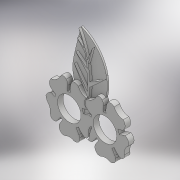
# Autodesk Inventor part: RosaV2
Saved by Autodesk Inventor 2017 (Build 210142000, 142)
## iProperties
Created: 2018-06-14
Part Number: RosaV2
Material: Generic
Document SubType Name: Modeling
Designer: Carolina Lema
Density: 1 g/cm^3
Appearance: Default
Author: Carolina Lema
Autodesk Inventor part; units mm, degrees
ref_plane "YZ Plane" through (0, 0, 0) normal (1, 0, 0) x (0, 1, 0)
ref_plane "XZ Plane" through (0, 0, 0) normal (0, 1, 0) x (-1, 0, 0)
ref_plane "XY Plane" through (0, 0, 0) normal (0, 0, 1) x (1, 0, 0)
sketch "Sketch1" plane through (0, 0, 0) normal (0, 1, 0) x (-1, 0, 0)
  arc A0 (-50.2935, -141.9625) -> (-50.5085, -138.2118) centre (-57.4787, -140.493) ccw
  arc A1 (-49.4604, -134.8668) -> (-50.5085, -138.2118) centre (-45.5145, -137.94) ccw
  arc A2 (-52.2706, -141.9093) -> (-53.5294, -134.3132) centre (-66.0628, -140.2926) ccw
  arc A3 (-60.8507, -147.4866) -> (-64.2809, -146.6761) centre (-66.0428, -161.7965) ccw
  circle A4 centre (-51.5636, -152.3854) radius 8.5
  arc A5 (-45.2271, -160.758) -> (-42.1345, -164.9104) centre (-15.6123, -141.9291) ccw
  arc A6 (-38.966, -164.9101) -> (-37.6707, -160.6686) centre (-43.0606, -161.3412) ccw
  arc A7 (-44.5421, -165.2935) -> (-46.8275, -161.7567) centre (-172.1244, -245.2288) ccw
  arc A8 (-37.8657, -145.4277) -> (-38.2191, -140.1494) centre (-41.6996, -143.0334) ccw
  arc A9 (-45.6096, -134.3885) -> (-38.2191, -140.1494) centre (-36.6467, -130.5112) ccw
  arc A10 (-36.1368, -156.274) -> (-37.6707, -160.6686) centre (-32.4682, -160.0194) ccw
  arc A11 (-36.1368, -156.274) -> (-34.6048, -152.385) centre (-42.1305, -151.6666) ccw
  arc A12 (-41.3682, -149.8747) -> (-38.503, -148.5121) centre (-47.6774, -132.9147) ccw
  arc A13 (-41.9398, -148.1863) -> (-37.8657, -145.4277) centre (-47.8277, -135.103) ccw
  arc A14 (-34.6048, -152.385) -> (-38.503, -148.5121) centre (-40.8573, -154.78) ccw
  arc A15 (-63.8657, -139.5775) -> (-58.174, -134.8668) centre (-65.1246, -132.2626) ccw
  arc A16 (-53.5294, -134.3132) -> (-58.174, -134.8668) centre (-55.4761, -137.7415) ccw
  arc A17 (-45.6096, -134.3885) -> (-49.4604, -134.8668) centre (-47.2959, -136.5525) ccw
  line L0 (-46.3394, -171.0352) -> (-46.3407, -171.0345)
  arc A18 (-48.8902, -170.6862) -> (-44.9412, -169.507) centre (-47.5666, -167.9168) ccw
  arc A19 (-65.6657, -161.3497) -> (-62.9245, -164.9101) centre (-62.7518, -161.9418) ccw
  arc A20 (-62.9245, -164.9101) -> (-58.2423, -160.4876) centre (-68.2851, -154.5449) ccw
  arc A21 (-56.5584, -161.6213) -> (-58.6246, -165.2834) centre (21.5695, -208.1162) ccw
  arc A22 (-58.6246, -165.2834) -> (-59.26, -166.6979) centre (-55.3426, -167.6077) ccw
  arc A23 (-59.26, -166.6979) -> (-53.816, -170.3276) centre (-55.8552, -167.4887) ccw
  arc A24 (-48.8902, -170.6862) -> (-53.816, -170.3276) centre (-51.7693, -176.2225) ccw
  arc A25 (-65.6657, -161.3497) -> (-67.4979, -155.3741) centre (-72.0774, -160.047) ccw
  arc A26 (-61.8781, -150.4206) -> (-66.2243, -148.9882) centre (-82.2432, -204.906) ccw
  arc A27 (-42.1345, -164.9104) -> (-38.966, -164.9101) centre (-40.5505, -161.8463) ccw
  arc A28 (-44.9412, -169.507) -> (-44.5421, -165.2935) centre (-48.2055, -167.0721) ccw
  arc A29 (-76.2935, -141.9625) -> (-76.5085, -138.2118) centre (-83.4787, -140.493) ccw
  arc A30 (-75.4604, -134.8668) -> (-76.5085, -138.2118) centre (-71.5145, -137.94) ccw
  arc A31 (-78.2706, -141.9093) -> (-79.5294, -134.3132) centre (-92.0628, -140.2926) ccw
  arc A32 (-86.8507, -147.4866) -> (-90.2809, -146.6761) centre (-92.0428, -161.7965) ccw
  circle A33 centre (-77.5636, -152.3854) radius 8.5
  arc A34 (-71.2271, -160.758) -> (-68.1345, -164.9104) centre (-41.6123, -141.9291) ccw
  arc A35 (-70.5421, -165.2935) -> (-72.8275, -161.7567) centre (-198.1244, -245.2288) ccw
  arc A36 (-63.8657, -145.4277) -> (-64.2191, -140.1494) centre (-67.6996, -143.0334) ccw
  arc A37 (-71.6096, -134.3885) -> (-64.2191, -140.1494) centre (-62.6467, -130.5112) ccw
  arc A38 (-67.9398, -148.1863) -> (-63.8657, -145.4277) centre (-73.8277, -135.103) ccw
  arc A39 (-90.7671, -139.6764) -> (-84.174, -134.8668) centre (-91.1246, -132.2626) ccw
  arc A40 (-79.5294, -134.3132) -> (-84.174, -134.8668) centre (-81.4761, -137.7415) ccw
  arc A41 (-71.6096, -134.3885) -> (-75.4604, -134.8668) centre (-73.2959, -136.5525) ccw
  line L1 (-72.3394, -171.0352) -> (-72.3407, -171.0345)
  arc A42 (-74.8902, -170.6862) -> (-70.9412, -169.507) centre (-73.5666, -167.9168) ccw
  arc A43 (-91.6657, -161.3497) -> (-88.9245, -164.9101) centre (-88.7518, -161.9418) ccw
  arc A44 (-88.9245, -164.9101) -> (-84.2423, -160.4876) centre (-94.2851, -154.5449) ccw
  arc A45 (-82.5584, -161.6213) -> (-84.6246, -165.2834) centre (-4.4305, -208.1162) ccw
  arc A46 (-84.6246, -165.2834) -> (-85.26, -166.6979) centre (-81.3426, -167.6077) ccw
  arc A47 (-85.26, -166.6979) -> (-79.816, -170.3276) centre (-81.8552, -167.4887) ccw
  arc A48 (-74.8902, -170.6862) -> (-79.816, -170.3276) centre (-77.7693, -176.2225) ccw
  arc A49 (-91.6639, -144.9966) -> (-90.2809, -146.6761) centre (-87.4857, -142.9652) ccw
  arc A50 (-90.7671, -139.6764) -> (-91.6639, -144.9966) centre (-87.4857, -142.9652) ccw
  arc A51 (-91.6657, -161.3497) -> (-94.028, -154.908) centre (-98.0774, -160.047) ccw
  arc A52 (-92.2243, -148.9882) -> (-94.028, -154.908) centre (-90.5316, -152.7386) ccw
  arc A53 (-87.8781, -150.4206) -> (-92.2243, -148.9882) centre (-108.2432, -204.906) ccw
  arc A54 (-68.1345, -164.9104) -> (-64.966, -164.9101) centre (-66.5505, -161.8463) ccw
  arc A55 (-70.9412, -169.507) -> (-70.5421, -165.2935) centre (-74.2055, -167.0721) ccw
  arc A56 (-66.2243, -148.9882) -> (-67.3918, -149.7806) centre (-64.5316, -152.7386) ccw
  circle A57 centre (-51.5636, -152.3854) radius 10.5
  circle A58 centre (-77.5636, -152.3854) radius 10.5
  arc A59 (-66.5505, -161.8463) -> (-64.966, -164.9101) centre (-62.3299, -161.6052) ccw
  arc A60 (-66.5505, -161.8463) -> (-67.9398, -156.5846) centre (-74.2403, -161.0624) ccw
  arc A61 (-64.2809, -146.6761) -> (-63.8657, -139.5775) centre (-67.8597, -142.9054) ccw
  line L2 (-53.5294, -134.3132) -> (-53.5294, -99.3132)
  line L3 (-53.5294, -99.3132) -> (-75.4604, -134.8668)
  line L4 (-75.4604, -134.8668) -> (-75.4604, -99.3132)
  line L5 (-75.4604, -99.3132) -> (-53.5294, -134.3132)
  point P0 (0, 0)
  point P1 (-51.4803, -152.4063)
  point P2 (-45.3977, -162.821)
  point P3 (-45.3977, -141.9574)
  point P4 (-33.5868, -132.2626)
  point P5 (-34.505, -161.7965)
  point P6 (-36.7472, -154.5449)
  point P7 (-47.2742, -170.9723)
  point P8 (-57.8397, -162.8189)
  point P9 (-56.1478, -170.9718)
  point P10 (-71.3977, -162.821)
  point P11 (-71.3977, -141.9574)
  point P12 (-59.5868, -132.2626)
  point P13 (-60.505, -161.7965)
  point P14 (-62.7472, -154.5449)
  point P15 (-73.2742, -170.9723)
  point P16 (-83.8397, -162.8189)
  point P17 (-82.1478, -170.9718)
  dimension "d2" = 21
  dimension "d3" = 21
  dimension "d0" = 17
  dimension "d1" = 17
  dimension "d6" = 35
  constraints: 128 point on circle, 60 centre point, 12 end point, 7 tangent, 2 coincident, 2 vertical, 1 concentric, 26 other
  measures "d0" diameter of A4
  measures "d1" diameter of A33
  measures "d6" distance of L2.start L2.end
extrude "Extrusion1" add sketch "Sketch1" along normal blind 4 contours A0 A1 A17 A9 A8 A13 A57 | A57 | A57 A3 A61 A15 A16 A2 | A12 A14 A11 A10 A6 A27 A5 A57 | A57 A20 A19 A25 A58 A56 A26 | A41 A37 A36 A38 A58 A29 A30 | A7 A28 A18 A24 A23 A22 A21 A57 | A58 | A58 A32 A49 A50 A39 A40 A31 | A60 A59 A54 A34 A58 | A58 A44 A43 A51 A52 A53 | A35 A55 A42 A48 A47 A46 A45 A58
sketch "Sketch4" plane through (0, 4, 0) normal (0, 1, 0) x (1, 0, 0)
  arc A0 (52.0058, 121.0973) -> (57.4996, 99.146) centre (415.9824, 200.5268) ccw
  arc A1 (54.1227, 139.9616) -> (52.0058, 121.0973) centre (80.9093, 127.4048) ccw
  arc A2 (63.864, 144.3907) -> (54.1227, 139.9616) centre (61.5923, 136.46) ccw
  arc A3 (57.4996, 99.146) -> (75.7221, 121.0973) centre (46.6692, 126.6758) ccw
  arc A4 (75.7221, 121.0973) -> (73.6052, 139.9616) centre (46.8187, 127.4048) ccw
  arc A5 (73.6052, 139.9616) -> (63.864, 144.3907) centre (66.1356, 136.46) ccw
  arc A6 (57.4996, 99.146) -> (63.864, 144.3907) centre (0.6464, 130.2132) ccw
  arc A7 (57.4996, 99.146) -> (62.7337, 144.6303) centre (-13.0806, 130.3112) ccw
  line L0 (63.5682, 139.1315) -> (54.1233, 123.015)
  line L1 (54.1233, 123.015) -> (63.864, 136.0011)
  line L2 (63.864, 124.6213) -> (55.2722, 115.1963)
  line L3 (55.2722, 115.1963) -> (63.5682, 121.4909)
  line L4 (61.2764, 109.723) -> (56.3279, 105.9683)
  line L5 (56.3279, 105.9683) -> (61.8855, 112.0649)
  line L6 (63.864, 116.0357) -> (67.3014, 107.1278)
  line L7 (67.3014, 107.1278) -> (64.3376, 118.3436)
  line L8 (65.3957, 132.4478) -> (75.743, 123.0153)
  line L9 (75.743, 123.0153) -> (65.424, 129.0627)
  point P0 (0, 0)
  constraints: 27 point on circle, 20 end point, 8 centre point, 2 parallel, 2 perpendicular, 2 tangent
extrude "Extrusion3" add sketch "Sketch4" against normal blind 1.2 contours A1 A2 A7 L0 L1 L2 L3 L5 L4 A0 | A6 L6 L7 L9 L8 A5 A4 A3
sketch "Sketch5" plane through (0, 4, 0) normal (0, 1, 0) x (1, 0, 0)
  arc A0 (65.3957, 132.4478) -> (64.6812, 140.0625) centre (0.6464, 130.2132) ccw projected
  circle A1 centre (51.5636, 152.3854) radius 8.5 projected
  circle A2 centre (77.5636, 152.3854) radius 8.5 projected
  arc A3 (63.8657, 139.5775) -> (63.5237, 139.5103) centre (65.1246, 132.2626) ccw projected
  arc A4 (63.4423, 140.1643) -> (63.8657, 139.5775) centre (67.8597, 142.9054) ccw projected
  arc A5 (63.4423, 140.1643) -> (62.8183, 144.1746) centre (-13.0806, 130.3112) ccw projected
  arc A6 (64.2809, 146.6761) -> (62.8183, 144.1746) centre (67.8597, 142.9054) ccw projected
  arc A7 (60.8507, 147.4866) -> (64.2809, 146.6761) centre (66.0428, 161.7965) ccw projected
  arc A8 (60.8507, 147.4866) -> (61.8781, 150.4206) centre (51.5636, 152.3854) ccw projected
  arc A9 (61.8781, 150.4206) -> (66.2243, 148.9882) centre (82.2432, 204.906) ccw projected
  arc A10 (66.2243, 148.9882) -> (67.3918, 149.7806) centre (64.5316, 152.7386) ccw projected
  arc A11 (67.3918, 149.7806) -> (67.9398, 148.1863) centre (77.5636, 152.3854) ccw projected
  arc A12 (67.9398, 148.1863) -> (63.8657, 145.4277) centre (73.8277, 135.103) ccw projected
  arc A13 (63.8657, 145.4277) -> (64.2191, 140.1494) centre (67.6996, 143.0334) ccw projected
  arc A14 (64.6812, 140.0625) -> (64.2191, 140.1494) centre (62.6467, 130.5112) ccw projected
  arc A15 (65.3957, 132.4478) -> (64.6812, 140.0625) centre (0.6464, 130.2132) ccw projected
  line L0 (65.3957, 132.4478) -> (75.743, 123.0153) projected
  line L1 (75.743, 123.0153) -> (65.424, 129.0627) projected
  arc A16 (64.3376, 118.3436) -> (65.424, 129.0627) centre (0.6464, 130.2132) ccw projected
  line L2 (64.3376, 118.3436) -> (67.3014, 107.1278) projected
  line L3 (67.3014, 107.1278) -> (63.864, 116.0357) projected
  arc A17 (57.4996, 99.146) -> (63.864, 116.0357) centre (0.6464, 130.2132) ccw projected
  arc A18 (57.4996, 99.146) -> (75.7221, 121.0973) centre (46.6692, 126.6758) ccw projected
  arc A19 (75.7221, 121.0973) -> (75.4494, 134.8528) centre (46.8187, 127.4048) ccw projected
  arc A20 (75.4494, 134.8528) -> (75.4604, 134.8668) centre (73.2959, 136.5525) ccw projected
  arc A21 (75.4604, 134.8668) -> (76.5085, 138.2118) centre (71.5145, 137.94) ccw projected
  arc A22 (76.2935, 141.9625) -> (76.5085, 138.2118) centre (83.4787, 140.493) ccw projected
  arc A23 (76.2935, 141.9625) -> (78.2706, 141.9093) centre (77.5636, 152.3854) ccw projected
  arc A24 (78.2706, 141.9093) -> (79.5294, 134.3132) centre (92.0628, 140.2926) ccw projected
  arc A25 (79.5294, 134.3132) -> (84.174, 134.8668) centre (81.4761, 137.7415) ccw projected
  arc A26 (90.7671, 139.6764) -> (84.174, 134.8668) centre (91.1246, 132.2626) ccw projected
  arc A27 (90.7671, 139.6764) -> (90.2809, 146.6761) centre (87.4857, 142.9652) ccw projected
  arc A28 (86.8507, 147.4866) -> (90.2809, 146.6761) centre (92.0428, 161.7965) ccw projected
  arc A29 (86.8507, 147.4866) -> (87.8781, 150.4206) centre (77.5636, 152.3854) ccw projected
  arc A30 (87.8781, 150.4206) -> (92.2243, 148.9882) centre (108.2432, 204.906) ccw projected
  arc A31 (92.2243, 148.9882) -> (94.028, 154.908) centre (90.5316, 152.7386) ccw projected
  arc A32 (91.6657, 161.3497) -> (94.028, 154.908) centre (98.0774, 160.047) ccw projected
  arc A33 (91.6657, 161.3497) -> (88.9245, 164.9101) centre (88.7518, 161.9418) ccw projected
  arc A34 (88.9245, 164.9101) -> (84.2423, 160.4876) centre (94.2851, 154.5449) ccw projected
  arc A35 (84.2423, 160.4876) -> (82.5584, 161.6213) centre (77.5636, 152.3854) ccw projected
  arc A36 (82.5584, 161.6213) -> (84.6246, 165.2834) centre (4.4305, 208.1162) ccw projected
  arc A37 (84.6246, 165.2834) -> (85.26, 166.6979) centre (81.3426, 167.6077) ccw projected
  arc A38 (85.26, 166.6979) -> (79.816, 170.3276) centre (81.8552, 167.4887) ccw projected
  arc A39 (74.8902, 170.6862) -> (79.816, 170.3276) centre (77.7693, 176.2225) ccw projected
  arc A40 (74.8902, 170.6862) -> (70.9412, 169.507) centre (73.5666, 167.9168) ccw projected
  arc A41 (70.9412, 169.507) -> (70.5421, 165.2935) centre (74.2055, 167.0721) ccw projected
  arc A42 (70.5421, 165.2935) -> (72.8275, 161.7567) centre (198.1244, 245.2288) ccw projected
  arc A43 (72.8275, 161.7567) -> (71.2271, 160.758) centre (77.5636, 152.3854) ccw projected
  arc A44 (71.2271, 160.758) -> (68.1345, 164.9104) centre (41.6123, 141.9291) ccw projected
  arc A45 (68.1345, 164.9104) -> (64.966, 164.9101) centre (66.5505, 161.8463) ccw projected
  arc A46 (66.5505, 161.8463) -> (64.966, 164.9101) centre (62.3299, 161.6052) ccw projected
  arc A47 (66.5505, 161.8463) -> (67.9398, 156.5846) centre (74.2403, 161.0624) ccw projected
  arc A48 (67.9398, 156.5846) -> (67.4979, 155.3741) centre (77.5636, 152.3854) ccw projected
  arc A49 (65.6657, 161.3497) -> (67.4979, 155.3741) centre (72.0774, 160.047) ccw projected
  arc A50 (65.6657, 161.3497) -> (62.9245, 164.9101) centre (62.7518, 161.9418) ccw projected
  arc A51 (62.9245, 164.9101) -> (58.2423, 160.4876) centre (68.2851, 154.5449) ccw projected
  arc A52 (58.2423, 160.4876) -> (56.5584, 161.6213) centre (51.5636, 152.3854) ccw projected
  arc A53 (56.5584, 161.6213) -> (58.6246, 165.2834) centre (-21.5695, 208.1162) ccw projected
  arc A54 (58.6246, 165.2834) -> (59.26, 166.6979) centre (55.3426, 167.6077) ccw projected
  arc A55 (59.26, 166.6979) -> (53.816, 170.3276) centre (55.8552, 167.4887) ccw projected
  arc A56 (48.8902, 170.6862) -> (53.816, 170.3276) centre (51.7693, 176.2225) ccw projected
  arc A57 (48.8902, 170.6862) -> (44.9412, 169.507) centre (47.5666, 167.9168) ccw projected
  arc A58 (44.9412, 169.507) -> (44.5421, 165.2935) centre (48.2055, 167.0721) ccw projected
  arc A59 (44.5421, 165.2935) -> (46.8275, 161.7567) centre (172.1244, 245.2288) ccw projected
  arc A60 (46.8275, 161.7567) -> (45.2271, 160.758) centre (51.5636, 152.3854) ccw projected
  arc A61 (45.2271, 160.758) -> (42.1345, 164.9104) centre (15.6123, 141.9291) ccw projected
  arc A62 (42.1345, 164.9104) -> (38.966, 164.9101) centre (40.5505, 161.8463) ccw projected
  arc A63 (38.966, 164.9101) -> (37.6707, 160.6686) centre (43.0606, 161.3412) ccw projected
  arc A64 (36.1368, 156.274) -> (37.6707, 160.6686) centre (32.4682, 160.0194) ccw projected
  arc A65 (36.1368, 156.274) -> (34.6048, 152.385) centre (42.1305, 151.6666) ccw projected
  arc A66 (34.6048, 152.385) -> (38.503, 148.5121) centre (40.8573, 154.78) ccw projected
  arc A67 (41.3682, 149.8747) -> (38.503, 148.5121) centre (47.6774, 132.9147) ccw projected
  arc A68 (41.3682, 149.8747) -> (41.9398, 148.1863) centre (51.5636, 152.3854) ccw projected
  arc A69 (41.9398, 148.1863) -> (37.8657, 145.4277) centre (47.8277, 135.103) ccw projected
  arc A70 (37.8657, 145.4277) -> (38.2191, 140.1494) centre (41.6996, 143.0334) ccw projected
  arc A71 (45.6096, 134.3885) -> (38.2191, 140.1494) centre (36.6467, 130.5112) ccw projected
  arc A72 (45.6096, 134.3885) -> (49.4604, 134.8668) centre (47.2959, 136.5525) ccw projected
  arc A73 (49.4604, 134.8668) -> (50.5085, 138.2118) centre (45.5145, 137.94) ccw projected
  arc A74 (50.2935, 141.9625) -> (50.5085, 138.2118) centre (57.4787, 140.493) ccw projected
  arc A75 (50.2935, 141.9625) -> (52.2706, 141.9093) centre (51.5636, 152.3854) ccw projected
  arc A76 (52.2706, 141.9093) -> (52.7297, 136.4107) centre (66.0628, 140.2926) ccw projected
  arc A77 (52.7297, 136.4107) -> (52.0058, 121.0973) centre (80.9093, 127.4048) ccw projected
  arc A78 (52.0058, 121.0973) -> (57.4996, 99.146) centre (415.9824, 200.5268) ccw projected
  arc A79 (57.4996, 99.146) -> (61.2764, 109.723) centre (-13.0806, 130.3112) ccw projected
  line L4 (61.2764, 109.723) -> (56.3279, 105.9683) projected
  line L5 (56.3279, 105.9683) -> (61.8855, 112.0649) projected
  arc A80 (61.8855, 112.0649) -> (63.5682, 121.4909) centre (-13.0806, 130.3112) ccw projected
  line L6 (63.5682, 121.4909) -> (55.2722, 115.1963) projected
  line L7 (55.2722, 115.1963) -> (63.864, 124.6213) projected
  arc A81 (63.864, 124.6213) -> (63.864, 136.0011) centre (-13.0806, 130.3112) ccw projected
  line L8 (63.864, 136.0011) -> (54.1233, 123.015) projected
  line L9 (54.1233, 123.015) -> (63.5682, 139.1315) projected
  arc A82 (63.5682, 139.1315) -> (63.5237, 139.5103) centre (-13.0806, 130.3112) ccw projected
  point P0 (0, 0)
extrude "Extrusion4" add sketch "Sketch5" against normal blind 3 contours L0 L1 A16 L2 L3 A17 A79 L4 L5 A80 L6 L7 A81 L8 L9 A82 A3 A4 A5 A6 A7 A8 A9 A10 A11 A12 A13 A14 A0
body "Solid1"
